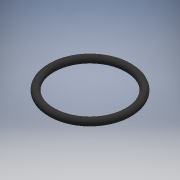
# Autodesk Inventor part: ORing_1x10mm
Saved by Autodesk Inventor 2018 (Build 220112000, 112)
## iProperties
Created: 2018-07-29
Part Number: ORing_1x10mm
Material: Rubber
Document SubType Name: Modeling
Designer: Bradley
Density: 0.93 g/cm^3
Appearance: Rubber - Black
Author: Bradley
Autodesk Inventor part; units mm, degrees
ref_plane "YZ Plane" through (0, 0, 0) normal (1, 0, 0) x (0, 1, 0)
ref_plane "XZ Plane" through (0, 0, 0) normal (0, 1, 0) x (-1, 0, 0)
ref_plane "XY Plane" through (0, 0, 0) normal (0, 0, 1) x (1, 0, 0)
sketch "Sketch1" plane through (0, 0, 0) normal (0, 1, 0) x (-1, 0, 0)
  circle A0 centre (-5.5, 0) radius 0.5
  line L0 (0, 0.5) -> (0, -0.5)
  line L1 (-5.5, 0.5) -> (-5.5, -0.5) construction
  point P0 (0, 0)
  point P1 (0, 0)
  dimension "d0" = 1
  dimension "d1" = 11
  constraints: 4 end point, 2 coincident, 2 midpoint, 2 point on circle, 2 vertical, 1 centre point, 1 horizontal alignment, 1 parallel
  measures "d0" diameter of A0
  measures "d1" diameter of A0.centre L0
revolve "Revolution1" add sketch "Sketch1" angle 360 about axis through (0, 0, 0.5) along (0, 0, -1)
body "Solid1"
